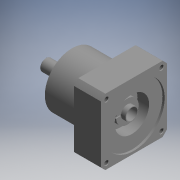
# Autodesk Inventor part: 552198 EMGA-120-P-G3-SAS-140---(P)
Saved by Autodesk Inventor 2017.3 (Build 213256000, 256)
## iProperties
Part Number: 552198 EMGA-120-P-G3-SAS-140---(P)
Material: Generic
Catalog Web Link: www.cadenas.de
Description: EMGA---(P)-gear unit
Vendor: FESTO
Document SubType Name: Modeling
Designer: partserver
Manufacturer: FESTO
Mass: 6000 g
Surface Area: 1205.08 cm^2
Volume: 1770.35 cm^3
Density: 1 g/cm^3
Appearance: PSOLRGB-175-175-175
Category: PARTsolutions
Company: FESTO
Title: 552198 EMGA-120-P-G3-SAS-140---(P)
Author: Cadenas PARTsolutions
Comments: gear unit
PSOL_IDENT_0: {$CADENAS_DATA\23d-libs\festo\parts\e\emga\emga.prj},213 {VTYP=3D},{NB=552198 EMGA-120-P-G3-SAS-140-
PSOL_IDENT_1: --(P)},{LINA=552198 EMGA-120-P-G3-SAS-140---(P)},{NN=EMGA---(P)},{DATE=23.11.2020 09:20:05},{GEOMDAT
PSOL_IDENT_2: E=19.11.2020 17:57:00},{VERSION=},{LINEID=190},{WBVAR=},{WBNUMERIC=}  {NB=552198 EMGA-120-P-G3-SAS-1
PSOL_IDENT_3: 40---(P)},{LINA=552198 EMGA-120-P-G3-SAS-140---(P)},{KT=DUMMY},{TNR=552198},{TYP=EMGA-120-P-G3-SAS-1
PSOL_IDENT_4: 40},{VER=10},{L=186.5},{L1=57.5},{L2=74.0},{L3=55},{L4=50},{L5=4},{L6=50.0},{L7=4.5},{L8=0},{L9=0},{
PSOL_IDENT_5: D1=25},{D2=35},{D3=80},{D4=130.0},{D5=24.00},{D6=100},{D7=185},{D8=165.0},{D9=115},{D10=0.0},{D11=48
PSOL_IDENT_6: .000},{D12=27.000},{D13=73.000},{L11=21.00},{L12=15.00},{L13=4.500},{L14=2.000},{D14=27.000},{B=140}
PSOL_IDENT_7: ,{B1=0.0},{T=0},{M=M10x16},{MA=10},{MTF=16},{M1=M10x25},{M1A=10},{M1TF=25},{L10=12.200},{CNSMASSEXAC
PSOL_IDENT_8: T=6.000}
NB: 552198 EMGA-120-P-G3-SAS-140---(P)
NN: EMGA---(P)
NT: gear unit
NBSYN: $TNR. $TYP.---(P)
LINA: 552198 EMGA-120-P-G3-SAS-140---(P)
CATALOG: Festo
TNR: 552198
TYP: EMGA-120-P-G3-SAS-140
CNSMASSEXACT: 6
SUPPLIER: FESTO
ARTICLENO: 552198 EMGA-120-P-G3-SAS-140---(P)
BOMINFO: 552198 EMGA-120-P-G3-SAS-140---(P)
CREATOR: CADENAS GmbH
Autodesk Inventor part; units mm, degrees
sketch "Sketch_1" plane through (0, 0, 0) normal (0, 0, 1) x (1, 0, 0)
  line L0 (55, 0) -> (-74, 0)
  line L1 (-74, 0) -> (-74, 57.5)
  line L2 (-74, 57.5) -> (0, 57.5)
  line L3 (0, 57.5) -> (0, 40)
  line L4 (0, 40) -> (4, 40)
  line L5 (4, 40) -> (4, 17.5)
  line L6 (4, 17.5) -> (5, 17.5)
  line L7 (5, 17.5) -> (5, 12.5)
  line L8 (5, 12.5) -> (54.5, 12.5)
  line L9 (54.5, 12.5) -> (55, 12)
  line L10 (55, 12) -> (55, 0)
  line L11 (55, 0) -> (-74, 0)
  constraints: 24 end point
revolve "Revolution1" add sketch "Sketch_1" angle 360 about axis through (55, 0, 0) along (1, 0, 0)
sketch "Sketch2" plane through (0, 0, 0) normal (1, 0, 0) x (0, 0, -1)
  point P0 (-35.3553, 35.3553)
hole "Hole1" at (0, 35.3553, 35.3553) direction (-1, 0, 0) diameter 8.376 depth 18 tip angle 120 countersink diameter 10 countersink angle 90 thread size "M10x1.5" class "6H" standard "ISO Metric profile"
sketch "Sketch3" plane through (0, 0, 0) normal (1, 0, 0) x (0, 0, -1)
  point P0 (-35.3553, -35.3553)
hole "Hole2" at (0, -35.3553, 35.3553) direction (-1, 0, 0) diameter 8.376 depth 18 tip angle 120 countersink diameter 10 countersink angle 90 thread size "M10x1.5" class "6H" standard "ISO Metric profile"
sketch "Sketch4" plane through (0, 0, 0) normal (1, 0, 0) x (0, 0, -1)
  point P0 (35.3553, 35.3553)
hole "Hole3" at (0, 35.3553, -35.3553) direction (-1, 0, 0) diameter 8.376 depth 18 tip angle 120 countersink diameter 10 countersink angle 90 thread size "M10x1.5" class "6H" standard "ISO Metric profile"
sketch "Sketch5" plane through (0, 0, 0) normal (1, 0, 0) x (0, 0, -1)
  point P0 (35.3553, -35.3553)
hole "Hole4" at (0, -35.3553, -35.3553) direction (-1, 0, 0) diameter 8.376 depth 18 tip angle 120 countersink diameter 10 countersink angle 90 thread size "M10x1.5" class "6H" standard "ISO Metric profile"
sketch "Sketch_13" plane through (-74, 0, 0) normal (1, 0, 0) x (0, 0, -1)
  arc A0 (-70, -60.4669) -> (-60.4669, -70) centre (0, 0) ccw
  line L0 (-60.4669, -70) -> (60.4669, -70)
  arc A1 (60.4669, -70) -> (70, -60.4669) centre (0, 0) ccw
  line L1 (70, -60.4669) -> (70, 60.4669)
  arc A2 (70, 60.4669) -> (60.4669, 70) centre (0, 0) ccw
  line L2 (60.4669, 70) -> (-60.4669, 70)
  arc A3 (-60.4669, 70) -> (-70, 60.4669) centre (0, 0) ccw
  line L3 (-70, 60.4669) -> (-70, -60.4669)
  constraints: 8 end point, 8 point on circle, 4 centre point
extrude "Extrusion1" add sketch "Sketch_13" against normal blind 57.5
sketch "Sketch_24" plane through (0, 0, 0) normal (0, 0, 1) x (1, 0, 0)
  line L0 (-81.5, 0) -> (-131.5, 0)
  line L1 (-131.5, 0) -> (-131.5, 65)
  line L2 (-131.5, 65) -> (-127, 65)
  line L3 (-127, 65) -> (-127, 36.5)
  line L4 (-127, 36.5) -> (-102.5, 36.5)
  line L5 (-102.5, 36.5) -> (-102.5, 24)
  line L6 (-102.5, 24) -> (-117.5, 24)
  line L7 (-117.5, 24) -> (-117.5, 13.5)
  line L8 (-117.5, 13.5) -> (-127, 13.5)
  line L9 (-127, 13.5) -> (-127, 12)
  line L10 (-127, 12) -> (-81.5, 12)
  line L11 (-81.5, 12) -> (-81.5, 0)
  line L12 (-81.5, 0) -> (-131.5, 0)
  constraints: 26 end point
revolve "Revolution2" cut sketch "Sketch_24" angle 360 about axis through (-81.5, 0, 0) along (1, 0, 0)
sketch "Sketch8" plane through (-131.5, 0, 0) normal (-1, 0, 0) x (0, 0, 1)
  point P0 (-58.3363, 58.3363)
hole "Hole5" at (-131.5, 58.3363, -58.3363) direction (1, 0, 0) diameter 8.376 depth 27 tip angle 120 countersink diameter 10 countersink angle 90 thread size "M10x1.5" class "6H" standard "ISO Metric profile"
sketch "Sketch9" plane through (-131.5, 0, 0) normal (-1, 0, 0) x (0, 0, 1)
  point P0 (-58.3363, -58.3363)
hole "Hole6" at (-131.5, -58.3363, -58.3363) direction (1, 0, 0) diameter 8.376 depth 27 tip angle 120 countersink diameter 10 countersink angle 90 thread size "M10x1.5" class "6H" standard "ISO Metric profile"
sketch "Sketch10" plane through (-131.5, 0, 0) normal (-1, 0, 0) x (0, 0, 1)
  point P0 (58.3363, 58.3363)
hole "Hole7" at (-131.5, 58.3363, 58.3363) direction (1, 0, 0) diameter 8.376 depth 27 tip angle 120 countersink diameter 10 countersink angle 90 thread size "M10x1.5" class "6H" standard "ISO Metric profile"
sketch "Sketch11" plane through (-131.5, 0, 0) normal (-1, 0, 0) x (0, 0, 1)
  point P0 (58.3363, -58.3363)
hole "Hole8" at (-131.5, -58.3363, 58.3363) direction (1, 0, 0) diameter 8.376 depth 27 tip angle 120 countersink diameter 10 countersink angle 90 thread size "M10x1.5" class "6H" standard "ISO Metric profile"
sketch "Sketch_19" plane through (-128, 0, 0) normal (1, 0, 0) x (0, 0, -1)
  line L0 (-1, -13.4629) -> (-1, -24)
  line L1 (-1, -24) -> (1, -24)
  line L2 (1, -24) -> (1, -13.4629)
  arc A0 (-1, -13.4629) -> (1, -13.4629) centre (0, 0) ccw
  constraints: 6 end point, 2 point on circle, 1 centre point
extrude "Extrusion2" cut sketch "Sketch_19" along normal blind 25.5
ref_plane "HGOANBAU_XY" through (0, 0, 0) normal (-1, 0, 0) x (0, 0, -1)
ref_plane "HGOANBAU_YZ" through (0, 0, 0) normal (0, 0, -1) x (0, -1, 0)
ref_plane "HGOANBAU_ZX" through (0, 0, 0) normal (0, -1, 0) x (-1, 0, 0)
ref_plane "S_1_XY" through (-143.7, 58.3363, -58.3363) normal (-1, 0, 0) x (0, 0, -1)
ref_plane "S_1_YZ" through (-143.7, 58.3363, -58.3363) normal (0, 0, -1) x (0, -1, 0)
ref_plane "S_1_ZX" through (-143.7, 58.3363, -58.3363) normal (0, -1, 0) x (-1, 0, 0)
ref_plane "S_2_XY" through (-143.7, 58.3363, 58.3363) normal (-1, 0, 0) x (0, 0, -1)
ref_plane "S_2_YZ" through (-143.7, 58.3363, 58.3363) normal (0, 0, -1) x (0, -1, 0)
ref_plane "S_2_ZX" through (-143.7, 58.3363, 58.3363) normal (0, -1, 0) x (-1, 0, 0)
ref_plane "S_3_XY" through (-143.7, -58.3363, 58.3363) normal (-1, 0, 0) x (0, 0, -1)
ref_plane "S_3_YZ" through (-143.7, -58.3363, 58.3363) normal (0, 0, -1) x (0, -1, 0)
ref_plane "S_3_ZX" through (-143.7, -58.3363, 58.3363) normal (0, -1, 0) x (-1, 0, 0)
ref_plane "S_4_XY" through (-143.7, -58.3363, -58.3363) normal (-1, 0, 0) x (0, 0, -1)
ref_plane "S_4_YZ" through (-143.7, -58.3363, -58.3363) normal (0, 0, -1) x (0, -1, 0)
ref_plane "S_4_ZX" through (-143.7, -58.3363, -58.3363) normal (0, -1, 0) x (-1, 0, 0)
body "Solid1"
